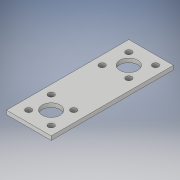
# Autodesk Inventor part: HolderV2
Saved by Autodesk Inventor 2019 (Build 230136000, 136)
## iProperties
Created: 2019-03-25
Part Number: HolderV2
Material: Ogólny
Document SubType Name: Modeling
Designer: atmat
Density: 1 g/cm^3
Appearance: Domyślna
Author: atmat
Autodesk Inventor part; units mm, degrees
ref_plane "YZ Plane" through (0, 0, 0) normal (1, 0, 0) x (0, 1, 0)
ref_plane "XZ Plane" through (0, 0, 0) normal (0, 1, 0) x (-1, 0, 0)
ref_plane "XY Plane" through (0, 0, 0) normal (0, 0, 1) x (1, 0, 0)
sketch "Szkic1" plane through (0, 0, 0) normal (0, 1, 0) x (-1, 0, 0)
  line L0 (11.2175, 30.7175) -> (-11.2175, 30.7175)
  line L1 (-11.2175, 30.7175) -> (-11.2175, -30.7175)
  line L2 (11.2175, -30.7175) -> (11.2175, 30.7175)
  circle A0 centre (6.7175, 12.7825) radius 1.5
  circle A1 centre (-6.7175, 26.2175) radius 1.5
  circle A2 centre (0, 19.5) radius 4.5
  circle A3 centre (0, -19.5) radius 4.5
  circle A4 centre (6.7175, -12.7825) radius 1.5
  circle A5 centre (-6.7175, -26.2175) radius 1.5
  circle A6 centre (5.6569, 25.1569) radius 1.5
  circle A7 centre (-5.6569, 13.8431) radius 1.5
  circle A8 centre (-5.6569, -13.8431) radius 1.5
  circle A9 centre (5.6569, -25.1569) radius 1.5
  line L3 (11.2175, -30.7175) -> (-11.2175, -30.7175)
  point P0 (0, 0)
  point P1 (0, 10.7072)
  dimension "d0" = 3
  dimension "d1" = 3
  dimension "d3" = 0
  dimension "d8" = 9
  dimension "d10" = 9
  dimension "d11" = 3
  dimension "d12" = 3
  dimension "d20" = 19.5
  dimension "d21" = 39
  dimension "d26" = 3
  dimension "d27" = 3
  dimension "d28" = 3
  dimension "d29" = 3
  dimension "d30" = 6.7175
  dimension "d31" = 6.7175
  dimension "d32" = 6.7175
  dimension "d33" = 6.7175
  dimension "d34" = 6.7175
  dimension "d35" = 6.7175
  dimension "d36" = 6.7175
  dimension "d37" = 6.7175
  dimension "d38" = 5.6569
  dimension "d39" = 5.6569
  dimension "d40" = 5.6569
  dimension "d41" = 5.6569
  dimension "d42" = 5.6569
  dimension "d43" = 5.6569
  dimension "d44" = 5.6569
  dimension "d45" = 5.6569
  dimension "d48" = 4.5
  dimension "d50" = 4.5
  dimension "d51" = 4.5
  dimension "d52" = 4.5
  constraints: 10 centre point, 8 end point, 2 horizontal, 1 parallel, 1 perpendicular
  measures "d0" diameter of A0
  measures "d1" diameter of A1
  measures "d3" horizontal distance of point (0, 10.707) point (0, 0)
  measures "d8" diameter of A2
  measures "d10" diameter of A3
  measures "d11" diameter of A4
  measures "d12" diameter of A5
  measures "d20" distance of point (0, 0) A2.centre
  measures "d21" distance of A3.centre A2.centre
  measures "d26" diameter of A6
  measures "d27" diameter of A7
  measures "d28" diameter of A8
  measures "d29" diameter of A9
  measures "d30" horizontal distance of A0.centre A2.centre
  measures "d31" horizontal distance of A0.centre A2.centre
  measures "d32" horizontal distance of A1.centre A2.centre
  measures "d33" horizontal distance of A1.centre A2.centre
  measures "d34" horizontal distance of A4.centre A3.centre
  measures "d35" horizontal distance of A4.centre A3.centre
  measures "d36" horizontal distance of A5.centre A3.centre
  measures "d37" horizontal distance of A3.centre A5.centre
  measures "d38" horizontal distance of A6.centre A2.centre
  measures "d39" horizontal distance of A6.centre A2.centre
  measures "d40" horizontal distance of A2.centre A7.centre
  measures "d41" horizontal distance of A2.centre A7.centre
  measures "d42" horizontal distance of A3.centre A8.centre
  measures "d43" horizontal distance of A3.centre A8.centre
  measures "d44" horizontal distance of A3.centre A9.centre
  measures "d45" horizontal distance of A3.centre A9.centre
  measures "d48" distance from line of A4.centre L2
  measures "d50" distance from line of L1 A1.centre
  measures "d51" distance from line of L0 A1.centre
  measures "d52" distance from line of L3 A5.centre
extrude "Wyciągnięcie proste1" add sketch "Szkic1" along normal blind 2
